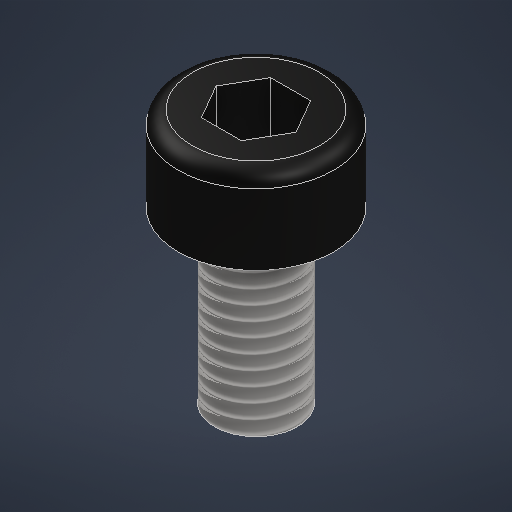
# Autodesk Inventor part: M3x16
Saved by Autodesk Inventor 2025.1 (Build 291241000, 241)
## iProperties
Created: 2024-10-26
Part Number: M3x16
Material: Generic
Document SubType Name: Modeling
Designer: jerem
Density: 1 g/cm^3
Appearance: Default
Author: jerem
Autodesk Inventor part; units mm, degrees
ref_plane "YZ Plane" through (0, 0, 0) normal (1, 0, 0) x (0, 1, 0)
ref_plane "XZ Plane" through (0, 0, 0) normal (0, 1, 0) x (-1, 0, 0)
ref_plane "XY Plane" through (0, 0, 0) normal (0, 0, 1) x (1, 0, 0)
sketch "Sketch1" plane through (0, 0, 0) normal (0, 1, 0) x (-1, 0, 0)
  circle A0 centre (0, 0) radius 1.465
  circle A1 centre (0, 0) radius 2.75
  line L0 (0.7073, -1.225) -> (-0.7073, -1.225)
  line L1 (-0.7073, -1.225) -> (-1.4145, 0)
  line L2 (-1.4145, 0) -> (-0.7073, 1.225)
  line L3 (-0.7073, 1.225) -> (0.7073, 1.225)
  line L4 (0.7073, 1.225) -> (1.4145, 0)
  line L5 (1.4145, 0) -> (0.7073, -1.225)
  dimension "d0" = 2.93
  dimension "d1" = 5.5
  dimension "d8" = 2.45
  constraints: 12 end point, 3 coincident, 2 centre point, 1 horizontal, 13 other
  measures "d0" diameter of A0
  measures "d1" diameter of A1
  measures "d8" distance between parallel lines of L3 L0
extrude "Extrusion1" add sketch "Sketch1" along normal blind 3 contours A0 | A1 | L0 L1 L2 L3 L4 L5
extrude "Extrusion2" add sketch "Sketch1" against normal blind 6 contours A0 | L0 L1 L2 L3 L4 L5
extrude "Extrusion3" cut sketch "Sketch1" against normal blind 2 from surface at 3 contours L0 L1 L2 L3 L4 L5
fillet "Fillet1" radius 0.5 1 edges at (2.75, 3, 0)
thread "Thread2" size "M3x0.5" class "6g" standard "ANSI Metric M Profile" full length
equation "\"d4\" = length"
equation "\"length\" = 6"
body "Solid1"
